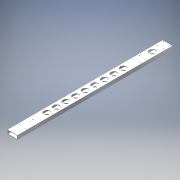
# Autodesk Inventor part: Sliding Extrusions
Saved by Autodesk Inventor 2019.4 (Build 234330000, 330)
## iProperties
Created: 2020-01-10
Part Number: Sliding Extrusions
Material: Aluminum 6061
Document SubType Name: Modeling
Designer: Mark
Mass: 1032.05 g
Surface Area: 2648.08 cm^2
Volume: 382.239 cm^3
Density: 2.7 g/cm^3
Appearance: Aluminum - Flat
Author: Mark
Autodesk Inventor part; units mm, degrees
ref_plane "YZ Plane" through (0, 0, 0) normal (1, 0, 0) x (0, 1, 0)
ref_plane "XZ Plane" through (0, 0, 0) normal (0, 1, 0) x (-1, 0, 0)
ref_plane "XY Plane" through (0, 0, 0) normal (0, 0, 1) x (1, 0, 0)
sketch "Sketch1" plane through (0, 0, 0) normal (0, 0, 1) x (1, 0, 0)
  line L0 (-30, -12.5) -> (30, -12.5)
  line L1 (30, -12.5) -> (30, 12.5)
  line L2 (30, 12.5) -> (-30, 12.5)
  line L3 (-30, 12.5) -> (-30, -12.5)
  line L4 (-30, -12.5) -> (30, 12.5) construction
  line L5 (30, -12.5) -> (-30, 12.5) construction
  line L6 (-27, -9.5) -> (27, -9.5)
  line L7 (27, -9.5) -> (27, 9.5)
  line L8 (27, 9.5) -> (-27, 9.5)
  line L9 (-27, 9.5) -> (-27, -9.5)
  line L10 (-27, -9.5) -> (27, 9.5) construction
  line L11 (27, -9.5) -> (-27, 9.5) construction
  point P0 (0, 0)
  dimension "d0" = 60
  dimension "d1" = 25
  dimension "d2" = 54
  dimension "d3" = 19
  constraints: 24 end point, 4 midpoint, 4 parallel, 2 horizontal, 2 perpendicular
  measures "d0" distance of L2.end L1.end
  measures "d1" distance of L1.end L0.end
  measures "d2" distance of L8.end L7.end
  measures "d3" distance of L7.end L6.end
extrude "Extrusion1" add sketch "Sketch1" along normal blind 970
sketch "Sketch2" plane through (-30, 12.5, 0) normal (0, 1, 0) x (1, 0, 0)
  circle A0 centre (50, -5) radius 2.75
  circle A1 centre (10, -5) radius 2.75
  circle A2 centre (10, -45) radius 2.75
  circle A3 centre (50, -45) radius 2.75
  line L0 (0, 0) -> (0, -970) projected
  line L1 (60, 0) -> (0, 0) projected
  circle A4 centre (50, -195) radius 2.75
  circle A5 centre (10, -195) radius 2.75
  circle A6 centre (10, -155) radius 2.75
  circle A7 centre (50, -155) radius 2.75
  circle A8 centre (10, -275) radius 2.75
  circle A9 centre (50, -275) radius 2.75
  circle A10 centre (50, -905) radius 2.75
  circle A11 centre (10, -905) radius 2.75
  line L2 (60, 0) -> (60, -970) projected
  line L3 (60, -970) -> (0, -970) projected
  point P0 (30, 0)
  dimension "d6" = 5.5
  dimension "d7" = 5.5
  dimension "d8" = 5.5
  dimension "d9" = 5.5
  dimension "d10" = 40
  dimension "d11" = 40
  dimension "d12" = 40
  dimension "d13" = 40
  dimension "d14" = 40
  dimension "d15" = 10
  dimension "d16" = 5
  dimension "d17" = 40
  dimension "d22" = 150
  dimension "d27" = 5.5
  dimension "d28" = 5.5
  dimension "d29" = 40
  dimension "d30" = 10
  dimension "d31" = 230
  dimension "d32" = 230
  dimension "d33" = 5.5
  dimension "d34" = 5.5
  dimension "d35" = 10
  dimension "d36" = 10
  dimension "d37" = 65
  dimension "d38" = 65
  constraints: 12 centre point, 1 vertical, 8 other
  measures "d6" diameter of A0
  measures "d7" diameter of A1
  measures "d8" diameter of A2
  measures "d9" diameter of A3
  measures "d10" horizontal distance of A1.centre A3.centre
  measures "d11" horizontal distance of A0.centre A2.centre
  measures "d12" distance of A0.centre A3.centre
  measures "d13" distance of A1.centre A2.centre
  measures "d14" horizontal distance of A1.centre A3.centre
  measures "d15" distance from line of L0 A1.centre
  measures "d16" distance from line of L1 A1.centre
  measures "d17" distance of A3.centre A2.centre
  measures "d22" distance of A3.centre A4.centre
  measures "d27" diameter of A8
  measures "d28" diameter of A9
  measures "d29" distance of A9.centre A8.centre
  measures "d30" distance from line of L0 A8.centre
  measures "d31" distance of A2.centre A8.centre
  measures "d32" distance of A3.centre A9.centre
  measures "d33" diameter of A10
  measures "d34" diameter of A11
  measures "d35" distance from line of L0 A11.centre
  measures "d36" distance from line of L2 A10.centre
  measures "d37" distance from line of L3 A10.centre
  measures "d38" distance from line of L3 A11.centre
extrude "Extrusion2" cut sketch "Sketch2" against normal blind 25 contours A0 | A1 | A2 | A3 | A4 | A5 | A6 | A7 | A8 | A9 | A10 | A11
sketch "Sketch3" plane through (30, -12.5, 0) normal (1, 0, 0) x (0, 0, -1)
  circle A0 centre (-854, 12.5) radius 2.75
  circle A1 centre (-840, 12.5) radius 2.75
  line L0 (0, 25) -> (-970, 25) projected
  line L1 (-970, 0) -> (-970, 25) projected
  circle A2 centre (-880, 12.5) radius 2.75
  circle A3 centre (-920, 12.5) radius 2.75
  point P0 (0, 12.5)
  dimension "d39" = 5.5
  dimension "d40" = 5.5
  dimension "d41" = 12.5
  dimension "d42" = 12.5
  dimension "d43" = 14
  dimension "d44" = 116
  dimension "d65" = 5.5
  dimension "d66" = 5.5
  dimension "d67" = 40
  dimension "d68" = 26
  dimension "d69" = 12.5
  dimension "d70" = 12.5
  constraints: 4 centre point
  measures "d39" diameter of A0
  measures "d40" diameter of A1
  measures "d41" distance from line of L0 A1.centre
  measures "d42" distance from line of L0 A0.centre
  measures "d43" distance of A1.centre A0.centre
  measures "d44" distance from line of L1 A0.centre
  measures "d65" diameter of A2
  measures "d66" diameter of A3
  measures "d67" distance of A2.centre A3.centre
  measures "d68" distance of A0.centre A2.centre
  measures "d69" distance from line of L0 A2.centre
  measures "d70" distance from line of L0 A3.centre
extrude "Extrusion3" cut sketch "Sketch3" against normal blind 60
sketch "Sketch4" plane through (-30, 12.5, 0) normal (0, 1, 0) x (1, 0, 0)
  circle A0 centre (25, -854) radius 2.75
  circle A1 centre (25, -837) radius 2.75
  line L0 (0, 0) -> (0, -970) projected
  line L1 (60, -970) -> (0, -970) projected
  circle A2 centre (30, -35) radius 20
  line L2 (60, 0) -> (0, 0) projected
  circle A3 centre (30, -95) radius 20
  circle A4 centre (30, -155) radius 20
  circle A5 centre (30, -215) radius 20
  circle A6 centre (30, -275) radius 20
  circle A7 centre (30, -335) radius 20
  circle A8 centre (30, -395) radius 20
  circle A9 centre (30, -455) radius 20
  circle A10 centre (30, -515) radius 20
  circle A11 centre (30, -575) radius 20
  circle A12 centre (30, -635) radius 20
  circle A13 centre (30, -695) radius 20
  circle A14 centre (30, -755) radius 20
  circle A15 centre (30, -815) radius 20
  circle A16 centre (30, -875) radius 20
  circle A17 centre (30, -935) radius 20
  point P0 (30, 0)
  dimension "d47" = 5.5
  dimension "d48" = 5.5
  dimension "d49" = 25
  dimension "d50" = 25
  dimension "d51" = 17
  dimension "d52" = 116
  dimension "d55" = 40
  dimension "d56" = 30
  dimension "d57" = 35
  dimension "d60" = 60
  constraints: 18 centre point, 1 vertical, 30 other
  measures "d47" diameter of A0
  measures "d48" diameter of A1
  measures "d49" distance from line of L0 A1.centre
  measures "d50" distance from line of L0 A0.centre
  measures "d51" distance of A0.centre A1.centre
  measures "d52" distance from line of L1 A0.centre
  measures "d55" diameter of A2
  measures "d56" distance from line of L0 A2.centre
  measures "d57" distance from line of L2 A2.centre
  measures "d60" distance of A2.centre A3.centre
extrude "Extrusion4" cut sketch "Sketch4" against normal blind 25 contours A0 A16 | A16 A0 | A1 A15 | A15 A1 | A3 | A6 | A7 | A8 | A9 | A10 | A11 | A12 | A13 | A14 picked at (24.9482, -854.1711) picked at (25.4594, -855.9294) picked at (24.6556, -837.9116) picked at (25.4907, -834.3679)
body "Solid1"
